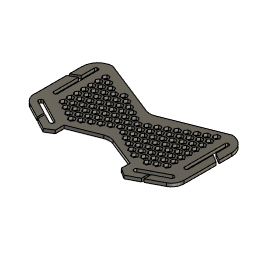
rear_adapter (Autodesk Fusion 360 design; units mm, degrees)
Autodesk Fusion 360 part; units mm, degrees
note: some values were not read from the file. Chosen so that the rebuilt part matches the saved one: which bodies a step acts on; which sketch regions a step uses.
(part 1 of 6)
sketch "Sketch1" plane through (0, 0, 0) normal (0, 0, 1) x (1, 0, 0)
  line L0 (235.0889, 171.2251) -> (235.0889, 121.2251)
  line L1 (165.0889, 121.2175) -> (165.0889, 171.2251)
  line L2 (200.0889, 189.725) -> (200.0889, 102.725) construction
  line L3 (235.0889, 121.2175) -> (235.0889, 171.2251)
  line L4 (165.0889, 121.2251) -> (165.0889, 171.2251)
  circle A0 centre (242.1889, 164.9963) radius 3.2
  circle A1 centre (242.1889, 127.4463) radius 3.2
  circle A2 centre (157.9889, 164.9963) radius 3.2
  circle A3 centre (157.9889, 127.4463) radius 3.2
  line L5 (165.0889, 146.2213) -> (235.0889, 146.2213) construction
  arc A4 (181.0338, 107.1206) -> (219.1356, 107.1166) centre (200.0889, 146.225) ccw
  line L6 (260.0889, 121.2175) -> (248.0889, 121.2175)
  line L7 (235.0889, 171.2251) -> (235.8524, 171.2251)
  line L8 (253.0889, 128.7175) -> (252.0889, 128.7175)
  line L9 (251.0889, 129.7175) -> (251.0889, 162.7175)
  line L10 (252.0889, 163.7175) -> (253.0889, 163.7175)
  line L11 (254.0889, 149.7175) -> (254.0889, 129.7175)
  arc A5 (254.0889, 162.7175) -> (253.0889, 163.7175) centre (253.0889, 162.7175) ccw
  arc A6 (252.0889, 163.7175) -> (251.0889, 162.7175) centre (252.0889, 162.7175) ccw
  arc A7 (253.0889, 128.7175) -> (254.0889, 129.7175) centre (253.0889, 129.7175) ccw
  arc A8 (251.0889, 129.7175) -> (252.0889, 128.7175) centre (252.0889, 129.7175) ccw
  line L12 (254.0889, 149.7175) -> (260.0889, 146.1766)
  line L13 (254.1214, 152.0206) -> (260.0889, 148.4989)
  line L14 (254.1214, 152.0206) -> (254.0889, 162.7175)
  line L15 (260.0889, 171.2251) -> (260.0889, 148.4989)
  line L16 (260.0889, 146.1766) -> (260.0889, 121.2175)
  arc A9 (146.0889, 129.7175) -> (147.0889, 128.7175) centre (147.0889, 129.7175) ccw
  line L17 (147.0889, 128.7175) -> (148.0889, 128.7175)
  arc A10 (148.0889, 128.7175) -> (149.0889, 129.7175) centre (148.0889, 129.7175) ccw
  line L18 (149.0889, 129.7175) -> (149.0889, 162.7175)
  line L19 (146.0889, 149.7175) -> (146.0889, 129.7175)
  line L20 (146.0889, 149.7175) -> (140.0889, 146.1766)
  line L21 (146.0563, 152.0206) -> (140.0889, 148.4989)
  line L22 (146.0563, 152.0206) -> (146.0889, 162.7175)
  arc A11 (147.0889, 163.7175) -> (146.0889, 162.7175) centre (147.0889, 162.7175) ccw
  line L23 (148.0889, 163.7175) -> (147.0889, 163.7175)
  arc A12 (149.0889, 162.7175) -> (148.0889, 163.7175) centre (148.0889, 162.7175) ccw
  line L24 (140.0889, 171.2251) -> (140.0889, 148.4989)
  line L25 (140.0889, 146.1766) -> (140.0889, 121.2251)
  line L26 (225.0889, 189.8602) -> (225.0889, 209.8602)
  line L27 (198.2466, 209.838) -> (175.0889, 209.838)
  line L28 (175.0889, 209.838) -> (175.0889, 189.6621)
  arc A13 (216.5899, 201.1843) -> (217.5889, 202.1852) centre (216.5889, 202.1843) ccw
  line L29 (217.5883, 202.8389) -> (217.5889, 202.1852)
  arc A14 (217.5883, 202.8389) -> (216.5883, 203.838) centre (216.5883, 202.838) ccw
  line L30 (196.5874, 203.838) -> (216.5883, 203.838)
  line L31 (196.5874, 203.838) -> (200.6627, 209.8351)
  line L32 (194.1849, 203.861) -> (198.3066, 209.9263)
  line L33 (194.1849, 203.861) -> (183.5873, 203.838)
  line L34 (216.5899, 201.1843) -> (183.5899, 201.1512)
  arc A15 (182.5889, 202.1503) -> (183.5899, 201.1512) centre (183.5889, 202.1512) ccw
  line L35 (182.5889, 202.1503) -> (182.5883, 202.8371)
  arc A16 (183.5873, 203.838) -> (182.5883, 202.8371) centre (183.5883, 202.838) ccw
  line L36 (200.6627, 209.8351) -> (225.0889, 209.8602)
  line L37 (190.0889, 193.451) -> (210.0889, 193.451)
  line L38 (211.0889, 192.451) -> (211.0889, 189.2169)
  line L39 (189.0889, 189.2169) -> (189.0889, 192.451)
  arc A17 (219.368, 185.3702) -> (211.82, 188.2537) centre (200.0889, 146.225) ccw
  arc A18 (188.3577, 188.2537) -> (180.8097, 185.3702) centre (200.0889, 146.225) ccw
  arc A19 (190.0889, 193.451) -> (189.0889, 192.451) centre (190.0889, 192.451) ccw
  arc A20 (211.0889, 192.451) -> (210.0889, 193.451) centre (210.0889, 192.451) ccw
  arc A21 (188.3577, 188.2537) -> (189.0889, 189.2169) centre (188.0889, 189.2169) ccw
  arc A22 (211.0889, 189.2169) -> (211.82, 188.2537) centre (212.0889, 189.2169) ccw
  line L40 (248.0889, 171.2251) -> (219.368, 185.3702)
  line L41 (225.0889, 189.8602) -> (260.0889, 171.2251)
  line L42 (248.0889, 171.2251) -> (235.8524, 171.2251)
  line L43 (248.0889, 121.2175) -> (219.1356, 107.1166)
  line L44 (260.0889, 121.2175) -> (223.2968, 101.9374)
  arc A23 (176.8737, 101.9412) -> (223.2968, 101.9374) centre (200.0889, 146.225) ccw
  line L45 (248.0889, 121.2175) -> (235.0889, 121.2175)
  line L46 (152.0889, 171.2251) -> (180.8097, 185.3702)
  line L47 (140.0889, 171.2251) -> (175.0889, 189.6621)
  line L48 (152.0889, 171.2251) -> (165.0889, 171.2251)
  line L49 (140.0889, 121.2251) -> (176.8737, 101.9412)
  line L50 (152.0889, 121.2251) -> (181.0338, 107.1206)
  line L51 (152.0889, 121.2251) -> (165.0889, 121.2175)
  point P0 (254.0889, 128.7175)
  point P1 (251.0889, 128.7175)
  point P2 (211.0889, 188.451)
  point P3 (189.0889, 188.451)
  dimension "d2" = 70
  dimension "d3" = 50
  dimension "d4" = 35
  dimension "d6" = 25
  dimension "d7" = 25
  dimension "d8" = 6.4
  dimension "d9" = 6.4
  dimension "d10" = 6.4
  dimension "d11" = 6.4
  dimension "d12" = 7.1
  dimension "d13" = 7.1
  dimension "d14" = 37.55
  dimension "d17" = 37.55
  dimension "d21" = 100
  dimension "d22" = 35
  dimension "d23" = 3
  dimension "d24" = 7.5
  dimension "d25" = 1
  dimension "d26" = 6
  dimension "d27" = 1
  dimension "d28" = 21
  dimension "d29" = 2
  dimension "d30" = 50
  dimension "d31" = 25
  dimension "d32" = 20
  dimension "d33" = 35
  dimension "d34" = 1
  dimension "d35" = 1
  dimension "d36" = 21
  dimension "d37" = 2
  dimension "d38" = 7.5
  dimension "d40" = 6
  dimension "d41" = 22
  dimension "d42" = 11
  dimension "d44" = 1
  dimension "d45" = 1
  dimension "d47" = 13
  dimension "d48" = 13
  dimension "d49" = 13
  dimension "d50" = 13
  constraint vertical L0
  constraint vertical L1
  constraint horizontal L7
  constraint vertical L15
  constraint horizontal L6
  constraint vertical L3
  constraint vertical L24
  constraint vertical L4
  constraint vertical A2.centre A3.centre
  constraint midpoint L1 L5.start
  constraint midpoint L3 L5.end
  constraint perpendicular L3 L5
  constraint concentric A4 A17
  constraint concentric A4 A23
  constraint coincident L40.start L7
  constraint horizontal L8
  constraint vertical L9
  constraint horizontal L10
  constraint vertical L11
  constraint tangent L11 A5
  constraint tangent L10 A5
  constraint tangent L9 A6
  constraint tangent L10 A6
  constraint equal A5 A6
  constraint coincident P0 L11
  constraint coincident P0 L8
  constraint tangent L11 A7
  constraint tangent L8 A7
  constraint equal A5 A7
  constraint coincident P1 L8
  constraint coincident P1 L9
  constraint tangent L8 A8
  constraint tangent L9 A8
  constraint coincident L12.end L15
  constraint parallel L12 L13
  constraint collinear L15 L16
  constraint symmetric L2 A5.start L22.end
  constraint symmetric L2 L10.end A11.start
  constraint symmetric L2 A5 A11
  constraint symmetric L2 L9.end L18.end
  constraint symmetric L2 L10.start L23.start
  constraint symmetric L2 A6 A12
  constraint symmetric L2 L11.end A9.start
  constraint symmetric L2 L8.start A9.end
  constraint symmetric L2 A7 A9
  constraint symmetric L2 L8.end L17.end
  constraint symmetric L2 L9.start A10.end
  constraint symmetric L2 A8 A10
  constraint symmetric L2 L11.start L19.start
  constraint symmetric L2 L12.end L20.end
  constraint symmetric L2 L13.start L21.start
  constraint symmetric L2 L13.end L21.end
  constraint collinear L24 L25
  constraint vertical L26
  constraint horizontal L27
  constraint vertical L28
  constraint tangent L30 A16
  constraint tangent L35 A16
  constraint tangent L34 A15
  constraint tangent A15 L35
  constraint equal A15 A16
  constraint tangent A14 L30
  constraint tangent L29 A14
  constraint equal A14 A16
  constraint tangent A13 L29
  constraint tangent A13 L34
  constraint parallel L31 L32
  constraint parallel L27 L30
  constraint coincident L32 L27.start
  constraint horizontal L37
  constraint vertical L38
  constraint vertical L39
  constraint coincident P3 A17
  constraint concentric A17 A18
  constraint tangent L39 A19
  constraint tangent L37 A19
  constraint tangent L37 A20
  constraint tangent L38 A20
  constraint equal A19 A20
  constraint coincident P3 L39
  constraint coincident P3 A18
  constraint tangent A18 A21
  constraint tangent L39 A21
  constraint equal A19 A21
  constraint coincident P2 L38
  constraint coincident P2 A17
  constraint tangent A17 A22
  constraint tangent L38 A22
  constraint tangent A17 L40
  constraint tangent A4 L43
  constraint tangent L44 A23
  constraint perpendicular L0 L45
  constraint tangent A18 L46
  constraint perpendicular L1 L48
  constraint tangent A23 L49
  constraint tangent A4 L50
  measures "d2" distance of L1.end L0.start
  measures "d3" distance of L0.start L0.end
  measures "d4" distance of L0 L2
  measures "d6" distance of L0.start L15.start
  measures "d7" distance of L1.end L24.start
  measures "d8" diameter of A2
  measures "d9" diameter of A3
  measures "d10" diameter of A0
  measures "d11" diameter of A1
  measures "d12" distance of L3 A1.centre
  measures "d13" distance of L4 A3.centre
  measures "d14" distance of A0.centre A1.centre
  measures "d17" distance of A2.centre A3.centre
  measures "d21" diameter of A23
  measures "d22" distance of L8 L10
  measures "d23" distance of P0 P1
  measures "d24" distance of L6 L8
  measures "d25" radius of A5
  measures "d26" distance of L11 L15
  measures "d27" radius of A8
  measures "d28" distance of L8 L11.start
  measures "d29" distance of L12 L13
  measures "d30" distance of L26.end L27.end
  measures "d31" distance of L2 L28
  measures "d32" distance of L26.start L26.end
  measures "d33" distance of L29 L35
  measures "d34" radius of A16
  measures "d35" radius of A13
  measures "d36" distance of L30.start L29
  measures "d37" distance of L31 L32
  measures "d38" distance of L26 A13.end
  measures "d40" distance of L27 L30
  measures "d41" distance of P2 P3
  measures "d42" distance of L2 L39
  measures "d44" radius of A19
  measures "d45" radius of A22
  measures "d47" distance of L0 L40.start
  measures "d48" distance of L3 L6.end
  measures "d49" distance of L1.end L46.start
  measures "d50" distance of L1 L50.start
extrude "Extrude1" add sketch "Sketch1" along normal blind 2.5 makes body 1
sketch "Sketch2" plane through (0, 0, 2.5) normal (0, 0, 1) x (-1, 0, 0)
  arc A0 (-181.0338, -107.1206) -> (-219.1356, -107.1166) centre (-200.0889, -146.225) ccw
  line L0 (-181.0338, -107.1206) -> (-152.0889, -121.2251)
  line L1 (-152.0889, -121.2251) -> (-165.0889, -121.2175)
  line L2 (-165.0889, -121.2175) -> (-165.0889, -171.2251)
  line L3 (-165.0889, -171.2251) -> (-152.0889, -171.2251)
  line L4 (-152.0889, -171.2251) -> (-180.8097, -185.3702)
  arc A1 (-188.3577, -188.2537) -> (-180.8097, -185.3702) centre (-200.0889, -146.225) ccw
  arc A2 (-188.3577, -188.2537) -> (-189.0889, -189.2169) centre (-188.0889, -189.2169) ccw
  line L5 (-189.0889, -189.2169) -> (-189.0889, -192.451)
  arc A3 (-190.0889, -193.451) -> (-189.0889, -192.451) centre (-190.0889, -192.451) ccw
  line L6 (-190.0889, -193.451) -> (-210.0889, -193.451)
  arc A4 (-211.0889, -192.451) -> (-210.0889, -193.451) centre (-210.0889, -192.451) ccw
  line L7 (-211.0889, -192.451) -> (-211.0889, -189.2169)
  arc A5 (-211.0889, -189.2169) -> (-211.82, -188.2537) centre (-212.0889, -189.2169) ccw
  arc A6 (-219.368, -185.3702) -> (-211.82, -188.2537) centre (-200.0889, -146.225) ccw
  line L8 (-219.368, -185.3702) -> (-248.0889, -171.2251)
  line L9 (-248.0889, -171.2251) -> (-235.0889, -171.2251)
  line L10 (-235.0889, -171.2251) -> (-235.0889, -121.2175)
  line L11 (-235.0889, -121.2175) -> (-248.0889, -121.2175)
  line L12 (-248.0889, -121.2175) -> (-219.1356, -107.1166)
  circle A7 centre (-242.1889, -127.4463) radius 3.2
  circle A8 centre (-157.9889, -164.9963) radius 3.2
  circle A9 centre (-157.9889, -127.4463) radius 3.2
  circle A10 centre (-242.1889, -164.9963) radius 3.2
  line L13 (-146.0889, -149.7175) -> (-140.0889, -146.1766)
  line L14 (-140.0889, -146.1766) -> (-140.0889, -121.2251)
  line L15 (-140.0889, -121.2251) -> (-176.8737, -101.9412)
  arc A11 (-176.8737, -101.9412) -> (-223.2968, -101.9374) centre (-200.0889, -146.225) ccw
  line L16 (-223.2968, -101.9374) -> (-260.0889, -121.2175)
  line L17 (-260.0889, -121.2175) -> (-260.0889, -146.1766)
  line L18 (-260.0889, -146.1766) -> (-254.0889, -149.7175)
  line L19 (-254.0889, -149.7175) -> (-254.0889, -129.7175)
  arc A12 (-253.0889, -128.7175) -> (-254.0889, -129.7175) centre (-253.0889, -129.7175) ccw
  line L20 (-253.0889, -128.7175) -> (-252.0889, -128.7175)
  arc A13 (-251.0889, -129.7175) -> (-252.0889, -128.7175) centre (-252.0889, -129.7175) ccw
  line L21 (-251.0889, -129.7175) -> (-251.0889, -162.7175)
  arc A14 (-252.0889, -163.7175) -> (-251.0889, -162.7175) centre (-252.0889, -162.7175) ccw
  line L22 (-252.0889, -163.7175) -> (-253.0889, -163.7175)
  arc A15 (-254.0889, -162.7175) -> (-253.0889, -163.7175) centre (-253.0889, -162.7175) ccw
  line L23 (-254.0889, -162.7175) -> (-254.1214, -152.0206)
  line L24 (-254.1214, -152.0206) -> (-260.0889, -148.4989)
  line L25 (-260.0889, -148.4989) -> (-260.0889, -171.2251)
  line L26 (-260.0889, -171.2251) -> (-225.0889, -189.8602)
  line L27 (-225.0889, -189.8602) -> (-225.0889, -209.8602)
  line L28 (-225.0889, -209.8602) -> (-200.6627, -209.8351)
  line L29 (-200.6627, -209.8351) -> (-196.5874, -203.838)
  line L30 (-196.5874, -203.838) -> (-216.5883, -203.838)
  arc A16 (-217.5883, -202.8389) -> (-216.5883, -203.838) centre (-216.5883, -202.838) ccw
  line L31 (-217.5883, -202.8389) -> (-217.5889, -202.1852)
  arc A17 (-216.5899, -201.1843) -> (-217.5889, -202.1852) centre (-216.5889, -202.1843) ccw
  line L32 (-216.5899, -201.1843) -> (-183.5899, -201.1512)
  arc A18 (-182.5889, -202.1503) -> (-183.5899, -201.1512) centre (-183.5889, -202.1512) ccw
  line L33 (-182.5889, -202.1503) -> (-182.5883, -202.8371)
  arc A19 (-183.5873, -203.838) -> (-182.5883, -202.8371) centre (-183.5883, -202.838) ccw
  line L34 (-183.5873, -203.838) -> (-194.1849, -203.861)
  line L35 (-194.1849, -203.861) -> (-198.2466, -209.838)
  line L36 (-198.2466, -209.838) -> (-175.0889, -209.838)
  line L37 (-175.0889, -209.838) -> (-175.0889, -189.6621)
  line L38 (-175.0889, -189.6621) -> (-140.0889, -171.2251)
  line L39 (-140.0889, -171.2251) -> (-140.0889, -148.4989)
  line L40 (-140.0889, -148.4989) -> (-146.0563, -152.0206)
  line L41 (-146.0563, -152.0206) -> (-146.0889, -162.7175)
  arc A20 (-147.0889, -163.7175) -> (-146.0889, -162.7175) centre (-147.0889, -162.7175) ccw
  line L42 (-147.0889, -163.7175) -> (-148.0889, -163.7175)
  arc A21 (-149.0889, -162.7175) -> (-148.0889, -163.7175) centre (-148.0889, -162.7175) ccw
  line L43 (-149.0889, -162.7175) -> (-149.0889, -129.7175)
  arc A22 (-148.0889, -128.7175) -> (-149.0889, -129.7175) centre (-148.0889, -129.7175) ccw
  line L44 (-148.0889, -128.7175) -> (-147.0889, -128.7175)
  arc A23 (-146.0889, -129.7175) -> (-147.0889, -128.7175) centre (-147.0889, -129.7175) ccw
  line L45 (-146.0889, -129.7175) -> (-146.0889, -149.7175)
  line L46 (-222.5842, -108.9932) -> (-222.5842, -101.5712)
  line L47 (-200.0889, -96.225) -> (-200.0842, -96.225)
  line L48 (-177.5842, -101.5759) -> (-177.5842, -108.9988)
  line L49 (-200.0842, -102.725) -> (-200.0842, -80) construction
  dimension "d55" = 22.5
  dimension "d62" = 22.5
  constraint vertical L46
  constraint horizontal L47
  constraint vertical L48
  constraint tangent A11 L47
  constraint midpoint A0 L49.start
  constraint perpendicular L47 L49
  constraint coincident A0 L48.end
  constraint coincident A0 L46.start
  constraint coincident A11 L46.end
  constraint coincident A11 L47.start
  constraint coincident L49 L47.end
  constraint coincident A11 L48.start
  measures "d55" distance of L46 L49
  measures "d62" distance of L48 L49
extrude "Extrude2" add sketch "Sketch2" along normal blind 4 contours A0 L0 L12 A11 L46 L47 L48 bodies 1
extrude "Extrude3" add 1 faces at (197.2054, 98.5357, 6.5) along direction (0, 0, -1) blind 10.5 separate body on bodies 1 makes body 2
sketch "Sketch3" plane through (0, 193.451, 0) normal (0, -1, 0) x (1, 0, 0)
  line L0 (190.0889, 0) -> (210.0889, 0)
  line L1 (210.0889, 0) -> (210.0889, 2.5)
  line L2 (210.0889, 2.5) -> (190.0889, 2.5)
  line L3 (190.0889, 2.5) -> (190.0889, 0)
  line L4 (184.5842, 5.75) -> (215.5842, 5.75)
  line L5 (217.5842, 3.75) -> (217.5842, -1.25)
  line L6 (215.5842, -3.25) -> (184.5842, -3.25)
  line L7 (182.5842, -1.25) -> (182.5842, 3.75)
  line L8 (200.0842, -0.8668) -> (200.0842, 23.75) construction
  line L9 (200.0842, 6.5) -> (200.0842, -4)
  line L10 (223.2968, 0) -> (176.8737, 0)
  arc A0 (184.5842, 5.75) -> (182.5842, 3.75) centre (184.5842, 3.75) ccw
  arc A1 (182.5842, -1.25) -> (184.5842, -3.25) centre (184.5842, -1.25) ccw
  arc A2 (217.5842, 3.75) -> (215.5842, 5.75) centre (215.5842, 3.75) ccw
  arc A3 (215.5842, -3.25) -> (217.5842, -1.25) centre (215.5842, -1.25) ccw
  point P0 (217.5842, 5.75)
  point P1 (217.5842, -3.25)
  dimension "d60" = 9
  dimension "d61" = 35
  dimension "d63" = 17.5
  dimension "d64" = 5.75
  dimension "d65" = 2
  constraint horizontal L4
  constraint vertical L5
  constraint horizontal L6
  constraint vertical L7
  constraint perpendicular L0 L8
  constraint coincident L8.end L9
  constraint tangent L7 A0
  constraint tangent L4 A0
  constraint tangent L7 A1
  constraint tangent L6 A1
  constraint equal A0 A1
  constraint coincident P0 L4
  constraint coincident P0 L5
  constraint tangent L4 A2
  constraint tangent L5 A2
  constraint equal A0 A2
  constraint coincident P1 L5
  constraint coincident P1 L6
  constraint tangent L5 A3
  constraint tangent L6 A3
  constraint equal A0 A3
  measures "d60" distance of P0 P1
  measures "d61" distance of L5 L7
  measures "d63" distance of L5 L8
  measures "d64" distance of L4 L10
  measures "d65" radius of A0
extrude "Extrude6" cut sketch "Sketch3" along normal blind 93 from surface at 10 bodies 2 1
extrude "Extrude4" add 1 faces at (197.2054, 98.5357, 6.5) along direction (0, 0, 1) blind 2 on bodies 2 bodies 2 1
extrude "Extrude5" add 1 faces at (197.2054, 98.5357, -4) along direction (0, 0, -1) blind 2 on bodies 2 bodies 2
fillet "Fillet1" radius 4 1 edges at (222.5842, 105.1837, 2.5) on bodies 2
fillet "Fillet2" radius 4 1 edges at (222.5842, 105.1837, 0) on bodies 2
fillet "Fillet3" radius 4 1 edges at (177.5842, 105.1887, 2.5) on bodies 2
fillet "Fillet4" radius 4 1 edges at (177.5842, 105.1887, 0) on bodies 2
fillet "Fillet5" radius 2 1 edges at (177.5842, 105.1887, 8.5) on bodies 2
fillet "Fillet6" radius 2 1 edges at (222.5842, 105.1837, 8.5) on bodies 2
fillet "Fillet7" radius 2 1 edges at (222.5842, 105.1837, -6) on bodies 2
fillet "Fillet8" radius 2 1 edges at (177.5842, 105.1887, -6) on bodies 2
sketch "Sketch4" plane through (0, 0, -6) normal (0, 0, -1) x (1, 0, 0)
  line L0 (179.5842, -100.6228) -> (179.5842, -107.8269)
  line L1 (179.5842, -107.8269) -> (181.0338, -107.1206)
  arc A0 (219.1356, -107.1166) -> (181.0338, -107.1206) centre (200.0889, -146.225) ccw
  line L2 (219.1356, -107.1166) -> (220.5842, -107.8221)
  line L3 (220.5842, -107.8221) -> (220.5842, -100.6186)
  arc A1 (220.5842, -100.6186) -> (200.0889, -96.225) centre (200.0889, -146.225) ccw
  line L4 (200.0889, -96.225) -> (200.0842, -96.225)
  arc A2 (200.0842, -96.225) -> (179.5842, -100.6228) centre (200.0889, -146.225) ccw
  line L5 (167.7861, -87.596) -> (228.8793, -87.596)
  line L6 (228.8793, -87.596) -> (228.8793, -121.9882)
  line L7 (228.8793, -121.9882) -> (167.7861, -121.9882)
  line L8 (167.7861, -121.9882) -> (167.7861, -87.596)
  constraint horizontal L5
  constraint vertical L6
  constraint horizontal L7
  constraint vertical L8
extrude "Extrude7" cut sketch "Sketch4" against normal blind 6 contours L0 L1 A0 L2 L3 A1 L4 A2 bodies 2
extrude "Extrude8" cut sketch "Sketch4" against normal blind 6 contours L0 L1 A0 L2 L3 A1 L4 A2 | L5 L6 L7 L8 bodies 2
fillet "Fillet9" radius 5 1 edges at (217.5842, 102.8921, 0) on bodies 2
fillet "Fillet10" radius 5 1 edges at (182.5842, 102.8958, 0) on bodies 2
sketch "Sketch5" plane through (0, 0, 2.5) normal (0, 0, 1) x (-1, 0, 0)
sketch "Sketch6" plane through (0, 0, 2.5) normal (0, 0, 1) x (-1, 0, 0)
  line L0 (-260.0889, -121.2175) -> (-260.0889, -114.4436)
  line L1 (-260.0889, -114.4436) -> (-232.4375, -99.9535)
  line L2 (-232.4375, -99.9535) -> (-226.5842, -103.6601)
  line L3 (-260.0889, -121.2175) -> (-223.2968, -101.9374)
  line L4 (-200, -80) -> (-200, -178.0194) construction
  line L5 (-139.9111, -121.2175) -> (-176.7032, -101.9374)
  line L6 (-167.5625, -99.9535) -> (-173.4158, -103.6601)
  line L7 (-139.9111, -114.4436) -> (-167.5625, -99.9535)
  line L8 (-139.9111, -121.2175) -> (-139.9111, -114.4436)
  point P0 (-260.0889, -121.2175)
  point P1 (-226.5842, -103.6601)
  dimension "d97" = 60
  dimension "d98" = 6
  constraint vertical L0
  constraint coincident P0 L0.start
  constraint coincident P1 L2.end
  constraint parallel L1 L3
  constraint vertical L4
  constraint symmetric P0 L4 L5.start
  constraint symmetric L0.end L4 L7.start
  constraint symmetric L1.end L4 L6.start
  constraint symmetric P1 L4 L6.end
  constraint symmetric L3.end L4 L5.end
  measures "d97" angle of L2 L3
  measures "d98" distance of L1 L3
extrude "Extrude9" add sketch "Sketch6" against normal blind 2.5 bodies 2 makes body 3 at (160.2964, 108.277, 2.5)
sketch "Sketch7" plane through (0, 0, 2.5) normal (0, 0, 1) x (-1, 0, 0)
  circle A0 centre (-242.1889, -164.9963) radius 3.2
  circle A1 centre (-157.9889, -127.4463) radius 3.2
  circle A2 centre (-157.9889, -164.9963) radius 3.2
  circle A3 centre (-242.1889, -127.4463) radius 3.2
  line L0 (-173.5842, -103.6656) -> (-173.5842, -110.7507)
  line L1 (-173.5842, -110.7507) -> (-152.0889, -121.2251)
  line L2 (-152.0889, -121.2251) -> (-165.0889, -121.2175)
  line L3 (-165.0889, -121.2175) -> (-165.0889, -171.2251)
  line L4 (-165.0889, -171.2251) -> (-152.0889, -171.2251)
  line L5 (-152.0889, -171.2251) -> (-180.8097, -185.3702)
  arc A4 (-188.3577, -188.2537) -> (-180.8097, -185.3702) centre (-200.0889, -146.225) ccw
  arc A5 (-188.3577, -188.2537) -> (-189.0889, -189.2169) centre (-188.0889, -189.2169) ccw
  line L6 (-189.0889, -189.2169) -> (-189.0889, -192.451)
  arc A6 (-190.0889, -193.451) -> (-189.0889, -192.451) centre (-190.0889, -192.451) ccw
  line L7 (-190.0889, -193.451) -> (-210.0889, -193.451)
  arc A7 (-211.0889, -192.451) -> (-210.0889, -193.451) centre (-210.0889, -192.451) ccw
  line L8 (-211.0889, -192.451) -> (-211.0889, -189.2169)
  arc A8 (-211.0889, -189.2169) -> (-211.82, -188.2537) centre (-212.0889, -189.2169) ccw
  arc A9 (-219.368, -185.3702) -> (-211.82, -188.2537) centre (-200.0889, -146.225) ccw
  line L9 (-219.368, -185.3702) -> (-248.0889, -171.2251)
  line L10 (-248.0889, -171.2251) -> (-235.0889, -171.2251)
  line L11 (-235.0889, -171.2251) -> (-235.0889, -121.2175)
  line L12 (-235.0889, -121.2175) -> (-248.0889, -121.2175)
  line L13 (-248.0889, -121.2175) -> (-226.5842, -110.7442)
  line L14 (-226.5842, -110.7442) -> (-226.5842, -103.6601)
  line L15 (-226.5842, -103.6601) -> (-232.4375, -99.9535)
  line L16 (-232.4375, -99.9535) -> (-260.0889, -114.4436)
  line L17 (-260.0889, -114.4436) -> (-260.0889, -146.1766)
  line L18 (-260.0889, -146.1766) -> (-254.0889, -149.7175)
  line L19 (-254.0889, -149.7175) -> (-254.0889, -129.7175)
  arc A10 (-253.0889, -128.7175) -> (-254.0889, -129.7175) centre (-253.0889, -129.7175) ccw
  line L20 (-253.0889, -128.7175) -> (-252.0889, -128.7175)
  arc A11 (-251.0889, -129.7175) -> (-252.0889, -128.7175) centre (-252.0889, -129.7175) ccw
  line L21 (-251.0889, -129.7175) -> (-251.0889, -162.7175)
  arc A12 (-252.0889, -163.7175) -> (-251.0889, -162.7175) centre (-252.0889, -162.7175) ccw
  line L22 (-252.0889, -163.7175) -> (-253.0889, -163.7175)
  arc A13 (-254.0889, -162.7175) -> (-253.0889, -163.7175) centre (-253.0889, -162.7175) ccw
  line L23 (-254.0889, -162.7175) -> (-254.1214, -152.0206)
  line L24 (-254.1214, -152.0206) -> (-260.0889, -148.4989)
  line L25 (-260.0889, -148.4989) -> (-260.0889, -171.2251)
  line L26 (-260.0889, -171.2251) -> (-225.0889, -189.8602)
  line L27 (-225.0889, -189.8602) -> (-225.0889, -209.8602)
  line L28 (-225.0889, -209.8602) -> (-200.6627, -209.8351)
  line L29 (-200.6627, -209.8351) -> (-196.5874, -203.838)
  line L30 (-196.5874, -203.838) -> (-216.5883, -203.838)
  arc A14 (-217.5883, -202.8389) -> (-216.5883, -203.838) centre (-216.5883, -202.838) ccw
  line L31 (-217.5883, -202.8389) -> (-217.5889, -202.1852)
  arc A15 (-216.5899, -201.1843) -> (-217.5889, -202.1852) centre (-216.5889, -202.1843) ccw
  line L32 (-216.5899, -201.1843) -> (-183.5899, -201.1512)
  arc A16 (-182.5889, -202.1503) -> (-183.5899, -201.1512) centre (-183.5889, -202.1512) ccw
  line L33 (-182.5889, -202.1503) -> (-182.5883, -202.8371)
  arc A17 (-183.5873, -203.838) -> (-182.5883, -202.8371) centre (-183.5883, -202.838) ccw
  line L34 (-183.5873, -203.838) -> (-194.1849, -203.861)
  line L35 (-194.1849, -203.861) -> (-198.2466, -209.838)
  line L36 (-198.2466, -209.838) -> (-175.0889, -209.838)
  line L37 (-175.0889, -209.838) -> (-175.0889, -189.6621)
  line L38 (-175.0889, -189.6621) -> (-140.0889, -171.2251)
  line L39 (-140.0889, -171.2251) -> (-140.0889, -148.4989)
  line L40 (-140.0889, -148.4989) -> (-146.0563, -152.0206)
  line L41 (-146.0563, -152.0206) -> (-146.0889, -162.7175)
  arc A18 (-147.0889, -163.7175) -> (-146.0889, -162.7175) centre (-147.0889, -162.7175) ccw
  line L42 (-147.0889, -163.7175) -> (-148.0889, -163.7175)
  arc A19 (-149.0889, -162.7175) -> (-148.0889, -163.7175) centre (-148.0889, -162.7175) ccw
  line L43 (-149.0889, -162.7175) -> (-149.0889, -129.7175)
  arc A20 (-148.0889, -128.7175) -> (-149.0889, -129.7175) centre (-148.0889, -129.7175) ccw
  line L44 (-148.0889, -128.7175) -> (-147.0889, -128.7175)
  arc A21 (-146.0889, -129.7175) -> (-147.0889, -128.7175) centre (-147.0889, -129.7175) ccw
  line L45 (-146.0889, -129.7175) -> (-146.0889, -149.7175)
  line L46 (-146.0889, -149.7175) -> (-140.0889, -146.1766)
  line L47 (-140.0889, -146.1766) -> (-140.0889, -121.2251)
  line L48 (-140.0889, -121.2251) -> (-173.5842, -103.6656)
  line L49 (-232.5206, -107.3354) -> (-232.343, -107.6745)
  line L50 (-232.9754, -109.6993) -> (-251.973, -119.6546)
  line L51 (-253.7746, -119.3399) -> (-254.0423, -119.0481)
  line L52 (-241.6644, -110.4336) -> (-241.6644, -104.7886)
  line L53 (-242.9644, -105.4699) -> (-242.9644, -111.1148)
  line L54 (-234.5455, -106.703) -> (-241.6644, -110.4336)
  line L55 (-242.9644, -111.1148) -> (-253.6331, -116.7055)
  arc A22 (-253.7746, -119.3399) -> (-251.973, -119.6546) centre (-252.6692, -118.326) ccw
  arc A23 (-253.6331, -116.7055) -> (-254.0423, -119.0481) centre (-252.9369, -118.0341) ccw
  arc A24 (-232.9754, -109.6993) -> (-232.343, -107.6745) centre (-233.6716, -108.3707) ccw
  arc A25 (-232.5206, -107.3354) -> (-234.5455, -106.703) centre (-233.8493, -108.0317) ccw
  line L56 (-200.0889, -189.725) -> (-200.0889, -102.725)
  line L57 (-167.6571, -107.3354) -> (-167.8348, -107.6745)
  arc A26 (-167.8348, -107.6745) -> (-167.2024, -109.6993) centre (-166.5061, -108.3707) ccw
  line L58 (-167.2024, -109.6993) -> (-148.2048, -119.6546)
  arc A27 (-148.2048, -119.6546) -> (-146.4031, -119.3399) centre (-147.5085, -118.326) ccw
  line L59 (-146.4031, -119.3399) -> (-146.1354, -119.0481)
  arc A28 (-146.1354, -119.0481) -> (-146.5446, -116.7055) centre (-147.2408, -118.0341) ccw
  line L60 (-157.2133, -111.1148) -> (-146.5446, -116.7055)
  line L61 (-157.2133, -105.4699) -> (-157.2133, -111.1148)
  line L62 (-158.5133, -110.4336) -> (-158.5133, -104.7886)
  line L63 (-165.6322, -106.703) -> (-158.5133, -110.4336)
  arc A29 (-165.6322, -106.703) -> (-167.6571, -107.3354) centre (-166.3285, -108.0317) ccw
  line L64 (-157.2133, -105.4699) -> (-157.2133, -104.8869)
  line L65 (-157.2133, -104.8869) -> (-158.5133, -104.1539)
  line L66 (-158.5133, -104.1539) -> (-158.5133, -104.7886)
  point P0 (-233.2169, -106.0068)
  point P1 (-255.3607, -117.6108)
  point P2 (-252.9948, -120.1901)
  dimension "d102" = 25
  dimension "d104" = 3.5
  dimension "d105" = 3.5
  dimension "d106" = 1.3
  dimension "d107" = 1.5
  dimension "d108" = 1.5
  dimension "d109" = 1.5
  dimension "d110" = 1.5
  dimension "d113" = 5
  constraint parallel L16 L54
  constraint perpendicular L49 L54
  constraint perpendicular L49 L50
  constraint coincident L16 L52.end
  constraint vertical L52
  constraint coincident L16 L53.start
  constraint coincident L53.end L54
  constraint parallel L52 L53
  constraint collinear L54 L55
  constraint coincident P2 L50
  constraint coincident P2 L51
  constraint tangent L50 A22
  constraint tangent L51 A22
  constraint coincident P1 L55
  constraint coincident P1 L51
  constraint tangent L55 A23
  constraint tangent L51 A23
  constraint tangent L50 A24
  constraint tangent L49 A24
  constraint coincident P0 L54
  constraint coincident P0 L49
  constraint tangent L54 A25
  constraint tangent L49 A25
  constraint symmetric L52.start L56 L62.start
  constraint symmetric L52.end L56 L62.end
  constraint symmetric L53.start L56 L61.start
  constraint symmetric L53.end L56 L60.start
  constraint symmetric L50.end L56 L58.end
  constraint symmetric L51.start L56 A27.end
  constraint symmetric A22 L56 A27
  constraint symmetric L55.end L56 A28.end
  constraint symmetric L51.end L56 L59.end
  constraint symmetric A23 L56 A28
  constraint symmetric L50.start L56 A26.end
  constraint symmetric L49.end L56 L57.end
  constraint symmetric A24 L56 A26
  constraint symmetric L54.start L56 L63.start
  constraint symmetric L49.start L56 L57.start
  constraint symmetric A25 L56 A29
  constraint parallel L61 L64
  constraint parallel L62 L66
  measures "d102" distance of P0 P1
  measures "d104" distance of L15.end L49
  measures "d105" distance of P1 P2
  measures "d106" distance of L52 L53
  measures "d107" radius of A22
  measures "d108" radius of A23
  measures "d109" radius of A24
  measures "d110" radius of A25
  measures "d113" distance of L16 L55
extrude "Extrude10" cut sketch "Sketch7" against normal blind 23 contours L48 A28 L60 L61 L62 L63 A29 L64 L65 L66 | L48 L57 A26 L58 A27 L59 A28 A29 | L16 L49 L50 L51 L52 L53 L54 L55 A22 A23 A24 A25 bodies 2 3 makes body 4 at (147.8897, 112.1753, 2.5)
extrude "Extrude11" add 1 faces at (169.3269, 105.8028, 1.6667) along direction (0.464159, 0.885752, 0) blind 0.6 on bodies 3 bodies 3 2
extrude "Extrude12" add 1 faces at (141.8561, 120.1983, 1.6667) along direction (0.464159, 0.885752, 0) blind 1.5 on bodies 4 bodies 4 3
extrude "Extrude13" cut 1 faces at (165.0889, 137.8867, 1.6667) along direction (-1, 0, 0) blind 1 on bodies 4 bodies 4
extrude "Extrude14" cut 1 faces at (235.0889, 137.8867, 0.8333) along direction (1, 0, 0) blind 1 on bodies 4 bodies 4
sketch "Sketch8" plane through (0, 0, 2.5) normal (0, 0, 1) x (-1, 0, 0)
  circle A0 centre (-242.1889, -127.4463) radius 3.2
  circle A1 centre (-157.9889, -127.4463) radius 3.2
  circle A2 centre (-242.1889, -164.9963) radius 3.2
  circle A3 centre (-157.9889, -164.9963) radius 3.2
  line L0 (-236.0889, -171.2251) -> (-236.0889, -121.2175)
  line L1 (-236.0889, -121.2175) -> (-248.0889, -121.2175)
  line L2 (-248.0889, -121.2175) -> (-226.5842, -110.7442)
  line L3 (-226.5842, -110.7442) -> (-226.5842, -103.6601)
  line L4 (-226.5842, -103.6601) -> (-232.4375, -99.9535)
  line L5 (-232.4375, -99.9535) -> (-241.6644, -104.7886)
  line L6 (-241.6644, -104.7886) -> (-241.6644, -110.4336)
  line L7 (-241.6644, -110.4336) -> (-234.5455, -106.703)
  arc A4 (-232.5206, -107.3354) -> (-234.5455, -106.703) centre (-233.8493, -108.0317) ccw
  line L8 (-232.5206, -107.3354) -> (-232.343, -107.6745)
  arc A5 (-232.9754, -109.6993) -> (-232.343, -107.6745) centre (-233.6716, -108.3707) ccw
  line L9 (-232.9754, -109.6993) -> (-251.973, -119.6546)
  arc A6 (-253.7746, -119.3399) -> (-251.973, -119.6546) centre (-252.6692, -118.326) ccw
  line L10 (-253.7746, -119.3399) -> (-254.0423, -119.0481)
  arc A7 (-253.6331, -116.7055) -> (-254.0423, -119.0481) centre (-252.9369, -118.0341) ccw
  line L11 (-253.6331, -116.7055) -> (-242.9644, -111.1148)
  line L12 (-242.9644, -111.1148) -> (-242.9644, -105.4699)
  line L13 (-242.9644, -105.4699) -> (-260.0889, -114.4436)
  line L14 (-260.0889, -114.4436) -> (-260.0889, -146.1766)
  line L15 (-260.0889, -146.1766) -> (-254.0889, -149.7175)
  line L16 (-254.0889, -149.7175) -> (-254.0889, -129.7175)
  arc A8 (-253.0889, -128.7175) -> (-254.0889, -129.7175) centre (-253.0889, -129.7175) ccw
  line L17 (-253.0889, -128.7175) -> (-252.0889, -128.7175)
  arc A9 (-251.0889, -129.7175) -> (-252.0889, -128.7175) centre (-252.0889, -129.7175) ccw
  line L18 (-251.0889, -129.7175) -> (-251.0889, -162.7175)
  arc A10 (-252.0889, -163.7175) -> (-251.0889, -162.7175) centre (-252.0889, -162.7175) ccw
  line L19 (-252.0889, -163.7175) -> (-253.0889, -163.7175)
  arc A11 (-254.0889, -162.7175) -> (-253.0889, -163.7175) centre (-253.0889, -162.7175) ccw
  line L20 (-254.0889, -162.7175) -> (-254.1214, -152.0206)
  line L21 (-254.1214, -152.0206) -> (-260.0889, -148.4989)
  line L22 (-260.0889, -148.4989) -> (-260.0889, -171.2251)
  line L23 (-260.0889, -171.2251) -> (-225.0889, -189.8602)
  line L24 (-225.0889, -189.8602) -> (-225.0889, -209.8602)
  line L25 (-225.0889, -209.8602) -> (-200.6627, -209.8351)
  line L26 (-200.6627, -209.8351) -> (-196.5874, -203.838)
  line L27 (-196.5874, -203.838) -> (-216.5883, -203.838)
  arc A12 (-217.5883, -202.8389) -> (-216.5883, -203.838) centre (-216.5883, -202.838) ccw
  line L28 (-217.5883, -202.8389) -> (-217.5889, -202.1852)
  arc A13 (-216.5899, -201.1843) -> (-217.5889, -202.1852) centre (-216.5889, -202.1843) ccw
  line L29 (-216.5899, -201.1843) -> (-183.5899, -201.1512)
  arc A14 (-182.5889, -202.1503) -> (-183.5899, -201.1512) centre (-183.5889, -202.1512) ccw
  line L30 (-182.5889, -202.1503) -> (-182.5883, -202.8371)
  arc A15 (-183.5873, -203.838) -> (-182.5883, -202.8371) centre (-183.5883, -202.838) ccw
  line L31 (-183.5873, -203.838) -> (-194.1849, -203.861)
  line L32 (-194.1849, -203.861) -> (-198.2466, -209.838)
  line L33 (-198.2466, -209.838) -> (-175.0889, -209.838)
  line L34 (-175.0889, -209.838) -> (-175.0889, -189.6621)
  line L35 (-175.0889, -189.6621) -> (-140.0889, -171.2251)
  line L36 (-140.0889, -171.2251) -> (-140.0889, -148.4989)
  line L37 (-140.0889, -148.4989) -> (-146.0563, -152.0206)
  line L38 (-146.0563, -152.0206) -> (-146.0889, -162.7175)
  arc A16 (-147.0889, -163.7175) -> (-146.0889, -162.7175) centre (-147.0889, -162.7175) ccw
  line L39 (-147.0889, -163.7175) -> (-148.0889, -163.7175)
  arc A17 (-149.0889, -162.7175) -> (-148.0889, -163.7175) centre (-148.0889, -162.7175) ccw
  line L40 (-149.0889, -162.7175) -> (-149.0889, -129.7175)
  arc A18 (-148.0889, -128.7175) -> (-149.0889, -129.7175) centre (-148.0889, -129.7175) ccw
  line L41 (-148.0889, -128.7175) -> (-147.0889, -128.7175)
  arc A19 (-146.0889, -129.7175) -> (-147.0889, -128.7175) centre (-147.0889, -129.7175) ccw
  line L42 (-146.0889, -129.7175) -> (-146.0889, -149.7175)
  line L43 (-146.0889, -149.7175) -> (-140.0889, -146.1766)
  line L44 (-140.0889, -146.1766) -> (-140.0889, -121.5567)
  line L45 (-140.0889, -121.5567) -> (-139.9111, -121.2175)
  line L46 (-139.9111, -121.2175) -> (-139.9111, -114.4436)
  line L47 (-139.9111, -114.4436) -> (-157.2133, -105.3767)
  line L48 (-157.2133, -105.3767) -> (-157.2133, -111.1148)
  line L49 (-157.2133, -111.1148) -> (-146.5446, -116.7055)
  arc A20 (-145.7461, -118.1598) -> (-146.5446, -116.7055) centre (-147.2408, -118.0341) ccw
  line L50 (-145.7461, -118.1598) -> (-146.3131, -119.2418)
  line L51 (-146.3131, -119.2418) -> (-146.4031, -119.3399)
  arc A21 (-148.2048, -119.6546) -> (-146.4031, -119.3399) centre (-147.5085, -118.326) ccw
  line L52 (-148.2048, -119.6546) -> (-167.2024, -109.6993)
  arc A22 (-167.8348, -107.6745) -> (-167.2024, -109.6993) centre (-166.5061, -108.3707) ccw
  line L53 (-167.8348, -107.6745) -> (-167.6652, -107.3509)
  line L54 (-167.6652, -107.3509) -> (-167.561, -107.4056)
  line L55 (-167.561, -107.4056) -> (-167.2825, -106.8741)
  arc A23 (-165.6322, -106.703) -> (-167.2825, -106.8741) centre (-166.3285, -108.0317) ccw
  line L56 (-165.6322, -106.703) -> (-158.5133, -110.4336)
  line L57 (-158.5133, -110.4336) -> (-158.5133, -104.6955)
  line L58 (-158.5133, -104.6955) -> (-167.5625, -99.9535)
  line L59 (-167.5625, -99.9535) -> (-173.4158, -103.6601)
  line L60 (-173.4158, -103.6601) -> (-173.4543, -103.7337)
  line L61 (-173.4543, -103.7337) -> (-173.5842, -103.6656)
  line L62 (-173.5842, -103.6656) -> (-173.5842, -110.7507)
  line L63 (-173.5842, -110.7507) -> (-152.0889, -121.2251)
  line L64 (-152.0889, -121.2251) -> (-164.0889, -121.2181)
  line L65 (-164.0889, -121.2181) -> (-164.0889, -171.2251)
  line L66 (-164.0889, -171.2251) -> (-152.0889, -171.2251)
  line L67 (-152.0889, -171.2251) -> (-180.8097, -185.3702)
  arc A24 (-188.3577, -188.2537) -> (-180.8097, -185.3702) centre (-200.0889, -146.225) ccw
  arc A25 (-188.3577, -188.2537) -> (-189.0889, -189.2169) centre (-188.0889, -189.2169) ccw
  line L68 (-189.0889, -189.2169) -> (-189.0889, -192.451)
  arc A26 (-190.0889, -193.451) -> (-189.0889, -192.451) centre (-190.0889, -192.451) ccw
  line L69 (-190.0889, -193.451) -> (-210.0889, -193.451)
  arc A27 (-211.0889, -192.451) -> (-210.0889, -193.451) centre (-210.0889, -192.451) ccw
  line L70 (-211.0889, -192.451) -> (-211.0889, -189.2169)
  arc A28 (-211.0889, -189.2169) -> (-211.82, -188.2537) centre (-212.0889, -189.2169) ccw
  arc A29 (-219.368, -185.3702) -> (-211.82, -188.2537) centre (-200.0889, -146.225) ccw
  line L71 (-219.368, -185.3702) -> (-248.0889, -171.2251)
  line L72 (-248.0889, -171.2251) -> (-236.0889, -171.2251)
  line L73 (-140.0889, -171.2251) -> (-262.7913, -171.2251)
  line L74 (-262.7913, -171.2251) -> (-262.7913, -224.0977)
  line L75 (-262.7913, -224.0977) -> (-140.0889, -224.0977)
  line L76 (-140.0889, -224.0977) -> (-140.0889, -171.2251)
  constraint horizontal L73
  constraint vertical L74
  constraint horizontal L75
  constraint vertical L76
  constraint coincident L35.end L36.start
extrude "Extrude15" cut sketch "Sketch8" along normal mid plane 60 contours L66 L67 A24 A25 L68 A26 L69 A27 L70 A28 A29 L71 L72 L73 | L23 L24 L25 L26 L27 A12 L28 A13 L29 A14 L30 A15 L31 L32 L33 L34 L35 L67 A24 A25 L68 A26 L69 A27 L70 A28 A29 L71 L73 | L23 L24 L25 L26 L27 A12 L28 A13 L29 A14 L30 A15 L31 L32 L33 L34 L35 L73 L74 L75 L76 bodies 4
sketch "Sketch9" plane through (0, 0, 2.5) normal (0, 0, 1) x (-1, 0, 0)
  line L0 (-260.0889, -171.2251) -> (-236.0889, -171.2251)
  line L1 (-236.0889, -171.2251) -> (-236.0889, -121.2175)
  line L2 (-236.0889, -121.2175) -> (-248.0889, -121.2175)
  line L3 (-248.0889, -121.2175) -> (-226.5842, -110.7442)
  line L4 (-226.5842, -110.7442) -> (-226.5842, -103.6601)
  line L5 (-226.5842, -103.6601) -> (-232.4375, -99.9535)
  line L6 (-232.4375, -99.9535) -> (-241.6644, -104.7886)
  line L7 (-241.6644, -104.7886) -> (-241.6644, -110.4336)
  line L8 (-241.6644, -110.4336) -> (-234.5455, -106.703)
  arc A0 (-232.5206, -107.3354) -> (-234.5455, -106.703) centre (-233.8493, -108.0317) ccw
  line L9 (-232.5206, -107.3354) -> (-232.343, -107.6745)
  arc A1 (-232.9754, -109.6993) -> (-232.343, -107.6745) centre (-233.6716, -108.3707) ccw
  line L10 (-232.9754, -109.6993) -> (-251.973, -119.6546)
  arc A2 (-253.7746, -119.3399) -> (-251.973, -119.6546) centre (-252.6692, -118.326) ccw
  line L11 (-253.7746, -119.3399) -> (-254.0423, -119.0481)
  arc A3 (-253.6331, -116.7055) -> (-254.0423, -119.0481) centre (-252.9369, -118.0341) ccw
  line L12 (-253.6331, -116.7055) -> (-242.9644, -111.1148)
  line L13 (-242.9644, -111.1148) -> (-242.9644, -105.4699)
  line L14 (-242.9644, -105.4699) -> (-260.0889, -114.4436)
  line L15 (-260.0889, -114.4436) -> (-260.0889, -146.1766)
  line L16 (-260.0889, -146.1766) -> (-254.0889, -149.7175)
  line L17 (-254.0889, -149.7175) -> (-254.0889, -129.7175)
  arc A4 (-253.0889, -128.7175) -> (-254.0889, -129.7175) centre (-253.0889, -129.7175) ccw
  line L18 (-253.0889, -128.7175) -> (-252.0889, -128.7175)
  arc A5 (-251.0889, -129.7175) -> (-252.0889, -128.7175) centre (-252.0889, -129.7175) ccw
  line L19 (-251.0889, -129.7175) -> (-251.0889, -162.7175)
  arc A6 (-252.0889, -163.7175) -> (-251.0889, -162.7175) centre (-252.0889, -162.7175) ccw
  line L20 (-252.0889, -163.7175) -> (-253.0889, -163.7175)
  arc A7 (-254.0889, -162.7175) -> (-253.0889, -163.7175) centre (-253.0889, -162.7175) ccw
  line L21 (-254.0889, -162.7175) -> (-254.1214, -152.0206)
  line L22 (-254.1214, -152.0206) -> (-260.0889, -148.4989)
  line L23 (-260.0889, -148.4989) -> (-260.0889, -171.2251)
  circle A8 centre (-242.1889, -164.9963) radius 3.2
  circle A9 centre (-242.1889, -127.4463) radius 3.2
  line L24 (-226.5842, -110.7442) -> (-173.5842, -110.7442)
  line L25 (-173.5842, -110.7442) -> (-173.5842, -92)
  line L26 (-173.5842, -92) -> (-226.5842, -92)
  line L27 (-226.5842, -92) -> (-226.5842, -110.7442)
  dimension "d124" = 53
  constraint horizontal L24
  constraint vertical L25
  constraint horizontal L26
  constraint vertical L27
  constraint coincident L3.end L4.start
  measures "d124" distance of L3.end L24.end
extrude "Extrude16" cut sketch "Sketch9" along normal mid plane 34 contours L4 L24 L25 L26 L27 bodies 4 makes body 5 at (245.3079, 140.673, 2.5)
sketch "Sketch10" plane through (0, 0, 2.5) normal (0, 0, 1) x (-1, 0, 0)
  line L0 (-260.0889, -171.2251) -> (-236.0889, -171.2251)
  line L1 (-236.0889, -171.2251) -> (-236.0889, -121.2175)
  line L2 (-236.0889, -121.2175) -> (-248.0889, -121.2175)
  line L3 (-248.0889, -121.2175) -> (-226.5842, -110.7442)
  line L4 (-226.5842, -110.7442) -> (-226.5842, -103.6601)
  line L5 (-226.5842, -103.6601) -> (-232.4375, -99.9535)
  line L6 (-232.4375, -99.9535) -> (-241.6644, -104.7886)
  line L7 (-241.6644, -104.7886) -> (-241.6644, -110.4336)
  line L8 (-241.6644, -110.4336) -> (-234.5455, -106.703)
  arc A0 (-232.5206, -107.3354) -> (-234.5455, -106.703) centre (-233.8493, -108.0317) ccw
  line L9 (-232.5206, -107.3354) -> (-232.343, -107.6745)
  arc A1 (-232.9754, -109.6993) -> (-232.343, -107.6745) centre (-233.6716, -108.3707) ccw
  line L10 (-232.9754, -109.6993) -> (-251.973, -119.6546)
  arc A2 (-253.7746, -119.3399) -> (-251.973, -119.6546) centre (-252.6692, -118.326) ccw
  line L11 (-253.7746, -119.3399) -> (-254.0423, -119.0481)
  arc A3 (-253.6331, -116.7055) -> (-254.0423, -119.0481) centre (-252.9369, -118.0341) ccw
  line L12 (-253.6331, -116.7055) -> (-242.9644, -111.1148)
  line L13 (-242.9644, -111.1148) -> (-242.9644, -105.4699)
  line L14 (-242.9644, -105.4699) -> (-260.0889, -114.4436)
  line L15 (-260.0889, -114.4436) -> (-260.0889, -146.1766)
  line L16 (-260.0889, -146.1766) -> (-254.0889, -149.7175)
  line L17 (-254.0889, -149.7175) -> (-254.0889, -129.7175)
  arc A4 (-253.0889, -128.7175) -> (-254.0889, -129.7175) centre (-253.0889, -129.7175) ccw
  line L18 (-253.0889, -128.7175) -> (-252.0889, -128.7175)
  arc A5 (-251.0889, -129.7175) -> (-252.0889, -128.7175) centre (-252.0889, -129.7175) ccw
  line L19 (-251.0889, -129.7175) -> (-251.0889, -162.7175)
  arc A6 (-252.0889, -163.7175) -> (-251.0889, -162.7175) centre (-252.0889, -162.7175) ccw
  line L20 (-252.0889, -163.7175) -> (-253.0889, -163.7175)
  arc A7 (-254.0889, -162.7175) -> (-253.0889, -163.7175) centre (-253.0889, -162.7175) ccw
  line L21 (-254.0889, -162.7175) -> (-254.1214, -152.0206)
  line L22 (-254.1214, -152.0206) -> (-260.0889, -148.4989)
  line L23 (-260.0889, -148.4989) -> (-260.0889, -171.2251)
  circle A8 centre (-242.1889, -164.9963) radius 3.2
  circle A9 centre (-242.1889, -127.4463) radius 3.2
extrude "Extrude17" add sketch "Sketch10" against normal up to surface (2.5 mm away) contours A8 | A9 bodies 5
sketch "Sketch11" plane through (0, 0, 0) normal (0, 0, -1) x (1, 0, 0)
  circle A0 centre (157.9889, -164.9963) radius 3.2
  circle A1 centre (157.9889, -127.4463) radius 3.2
  line L0 (173.5975, -110.7442) -> (173.5842, -110.7442)
  line L1 (173.5842, -110.7442) -> (173.5842, -103.6656)
  line L2 (173.5842, -103.6656) -> (173.4543, -103.7337)
  line L3 (173.4543, -103.7337) -> (173.4158, -103.6601)
  line L4 (173.4158, -103.6601) -> (167.5625, -99.9535)
  line L5 (167.5625, -99.9535) -> (158.5133, -104.6955)
  line L6 (158.5133, -104.6955) -> (158.5133, -110.4336)
  line L7 (158.5133, -110.4336) -> (165.6322, -106.703)
  arc A2 (167.2825, -106.8741) -> (165.6322, -106.703) centre (166.3285, -108.0317) ccw
  line L8 (167.2825, -106.8741) -> (167.561, -107.4056)
  line L9 (167.561, -107.4056) -> (167.6652, -107.3509)
  line L10 (167.6652, -107.3509) -> (167.8348, -107.6745)
  arc A3 (167.2024, -109.6993) -> (167.8348, -107.6745) centre (166.5061, -108.3707) ccw
  line L11 (167.2024, -109.6993) -> (148.2048, -119.6546)
  arc A4 (146.4031, -119.3399) -> (148.2048, -119.6546) centre (147.5085, -118.326) ccw
  line L12 (146.4031, -119.3399) -> (146.3131, -119.2418)
  line L13 (146.3131, -119.2418) -> (145.7461, -118.1598)
  arc A5 (146.5446, -116.7055) -> (145.7461, -118.1598) centre (147.2408, -118.0341) ccw
  line L14 (146.5446, -116.7055) -> (157.2133, -111.1148)
  line L15 (157.2133, -111.1148) -> (157.2133, -105.3767)
  line L16 (157.2133, -105.3767) -> (139.9111, -114.4436)
  line L17 (139.9111, -114.4436) -> (139.9111, -121.2175)
  line L18 (139.9111, -121.2175) -> (140.0889, -121.5567)
  line L19 (140.0889, -121.5567) -> (140.0889, -146.1766)
  line L20 (140.0889, -146.1766) -> (146.0889, -149.7175)
  line L21 (146.0889, -149.7175) -> (146.0889, -129.7175)
  arc A6 (147.0889, -128.7175) -> (146.0889, -129.7175) centre (147.0889, -129.7175) ccw
  line L22 (147.0889, -128.7175) -> (148.0889, -128.7175)
  arc A7 (149.0889, -129.7175) -> (148.0889, -128.7175) centre (148.0889, -129.7175) ccw
  line L23 (149.0889, -129.7175) -> (149.0889, -162.7175)
  arc A8 (148.0889, -163.7175) -> (149.0889, -162.7175) centre (148.0889, -162.7175) ccw
  line L24 (148.0889, -163.7175) -> (147.0889, -163.7175)
  arc A9 (146.0889, -162.7175) -> (147.0889, -163.7175) centre (147.0889, -162.7175) ccw
  line L25 (146.0889, -162.7175) -> (146.0563, -152.0206)
  line L26 (146.0563, -152.0206) -> (140.0889, -148.4989)
  line L27 (140.0889, -148.4989) -> (140.0889, -171.2251)
  line L28 (140.0889, -171.2251) -> (164.0889, -171.2251)
  line L29 (164.0889, -171.2251) -> (164.0889, -121.2181)
  line L30 (164.0889, -121.2181) -> (152.0889, -121.2251)
  line L31 (152.0889, -121.2251) -> (173.5975, -110.7442)
  line L32 (164.0889, -121.2181) -> (152.0889, -121.2181)
  line L33 (152.0889, -121.2181) -> (152.0889, -171.2251)
  line L34 (152.0889, -171.2251) -> (164.0889, -171.2251)
  line L35 (164.0889, -171.2251) -> (164.0889, -121.2181)
  constraint horizontal L32
  constraint vertical L33
  constraint horizontal L34
  constraint vertical L35
  constraint midpoint L28 L33.end
  constraint coincident L29.end L30.start
extrude "Extrude18" add sketch "Sketch11" against normal up to surface (2.5 mm away) contours A0 | A1 bodies 4